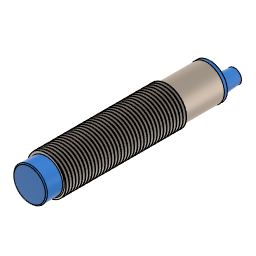
Inductive Proximity Sensor LJ12A3-4-Z_BX (Autodesk Fusion 360 design; units mm, degrees)
Autodesk Fusion 360 part; units mm, degrees
sketch "Sketch1" plane through (0, 0, 0) normal (0, 1, 0) x (1, 0, 0)
  circle A0 centre (0, 0) radius 5.15
  dimension "d1" = 10.3
  constraint coincident A0.centre origin
  measures "d1" diameter of A0
extrude "Extrude1" add sketch "Sketch1" along normal blind 5 makes body 1
sketch "Sketch2" plane through (0, 5, 0) normal (0, 1, 0) x (-1, 0, 0)
  circle A0 centre (0, 0) radius 5.15
  circle A1 centre (0, 0) radius 6
  dimension "d4" = 12
  constraint coincident A0.centre A1.centre
  measures "d4" diameter of A1
extrude "Extrude2" add sketch "Sketch2" along normal blind 37.5 separate body contours A0 | A1 makes body 2
sketch "Sketch3" plane through (0, 42.5, 0) normal (0, 1, 0) x (-1, 0, 0)
  circle A0 centre (0, 0) radius 6
  circle A1 centre (0, 0) radius 5.4
  dimension "d7" = 10.8
  constraint coincident A0.centre A1.centre
  measures "d7" diameter of A1
extrude "Extrude3" add sketch "Sketch3" along normal blind 12 separate body contours A1 makes body 3
sketch "Sketch4" plane through (0, 54.5, 0) normal (0, 1, 0) x (-1, 0, 0)
  circle A0 centre (0, 0) radius 5.4
extrude "Extrude4" add sketch "Sketch4" along normal blind 1 separate body makes body 4
thread "Thread1" "ISO Metric profile 12.0 M12x1 6g" major diameter 11.884 minor diameter 10.7405 pitch 1 angle 60 modelled right hand crest width 0.1426 on face at (-5.9925, 30, -0.2991) crest through (-5.942, 4.75, 0) on bodies 2
combine "Combine1" operation add target body 2 tool bodies 3
sketch "Sketch5" plane through (0, 55.5, 0) normal (0, 1, 0) x (-1, 0, 0)
  circle A0 centre (0, 0) radius 5.4
  circle A1 centre (-2.5, 0) radius 2.5
  dimension "d12" = 5
  measures "d12" diameter of A1
extrude "Extrude5" add sketch "Sketch5" along normal blind 5 draft -4 contours A1 bodies 4
sketch "Sketch6" plane through (0, 55.5, 0) normal (0, 1, 0) x (-1, 0, 0)
  circle A0 centre (-2.5, 0) radius 2.5
  circle A1 centre (0, 0) radius 5.4
  circle A2 centre (3, 0) radius 1
  dimension "d15" = 2
  measures "d15" diameter of A2
extrude "Extrude6" add sketch "Sketch6" along normal blind 0.3 separate body contours A2 makes body 5
fillet "Fillet1" radius 1 1 edges at (-2.0677, 55.8, -0.3616) on bodies 5
fillet "Fillet2" radius 0.1 1 edges at (5.0346, 55.5, -1.9527) on bodies 4
fillet "Fillet3" radius 0.3 1 edges at (-4.8015, 0, 1.8623) on bodies 1
